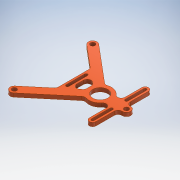
# Autodesk Inventor part: Pok Mk3 Base
Saved by Autodesk Inventor 2018.2 (Build 222227000, 227)
## iProperties
Created: 2018-02-12
Part Number: Pok Mk3 Base
Material: ABS Plastic
Document SubType Name: Modeling
Designer: Moochster
Density: 1.06 g/cm^3
Appearance: Smooth - Light Orange
Author: Moochster
Autodesk Inventor part; units mm, degrees
ref_plane "YZ Plane" through (0, 0, 0) normal (1, 0, 0) x (0, 1, 0)
ref_plane "XZ Plane" through (0, 0, 0) normal (0, 1, 0) x (-1, 0, 0)
ref_plane "XY Plane" through (0, 0, 0) normal (0, 0, 1) x (1, 0, 0)
sketch "Sketch1" plane through (0, 0, 0) normal (0, 0, 1) x (1, 0, 0)
  arc A0 (-5.6292, 10.5978) -> (-11.4143, 3.7034) centre (0, 0) ccw
  line L0 (11.1243, -4.5) -> (28, -4.5)
  arc A1 (28, -4.5) -> (28, 4.5) centre (28, 0) ccw
  line L1 (28, 4.5) -> (11.1243, 4.5)
  line L2 (0, 0) -> (28, 0) construction
  line L3 (0, 0) -> (-49.7929, 41.7812) construction
  line L4 (-5.6292, 10.5978) -> (-46.9003, 45.2284)
  arc A2 (-46.9003, 45.2284) -> (-52.6854, 38.334) centre (-49.7929, 41.7812) ccw
  line L5 (-52.6854, 38.334) -> (-11.4143, 3.7034)
  arc A3 (11.1243, 4.5) -> (-5.6292, 10.5978) centre (0, 0) ccw
  arc A4 (-11.4143, 3.7034) -> (-11.4143, -3.7034) centre (0, 0) ccw
  line L6 (-5.6292, -10.5978) -> (-46.9003, -45.2284)
  arc A5 (-52.6854, -38.334) -> (-46.9003, -45.2284) centre (-49.7929, -41.7812) ccw
  line L7 (-52.6854, -38.334) -> (-11.4143, -3.7034)
  arc A6 (-5.6292, -10.5978) -> (11.1243, 4.5) centre (0, 0) ccw
  arc A7 (-11.4143, -3.7034) -> (-5.6292, -10.5978) centre (0, 0) ccw
  circle A8 centre (28, 0) radius 2.5
  circle A9 centre (-49.7929, 41.7812) radius 2.5
  circle A10 centre (-49.7929, -41.7812) radius 2.5
  circle A11 centre (0, 0) radius 8.0875
  dimension "d0" = 24
  dimension "d5" = 5
  dimension "d6" = 2
  dimension "d7" = 28
  dimension "d8" = 65
  dimension "d9" = 140
  dimension "d10" = 5
  dimension "d11" = 2
  dimension "d12" = 5
  dimension "d13" = 16.175
  constraints: 19 point on circle, 16 end point, 12 centre point, 5 coincident, 5 symmetric about line, 4 parallel, 4 tangent, 1 horizontal, 1 other
  measures "d0" diameter of A0
  measures "d5" diameter of A8
  measures "d6" radial gap between concentric circles of A1 A8
  measures "d7" distance of L2.start L2.end
  measures "d8" distance of L2.start L3.end
  measures "d9" angle of L2 L3
  measures "d10" diameter of A9
  measures "d11" radial gap between concentric circles of A2 A9
  measures "d12" diameter of A10
  measures "d13" diameter of A11
extrude "Extrusion2" add sketch "Sketch1" along normal blind 4
sketch "Sketch2" plane through (0, 0, 0) normal (0, 0, 1) x (1, 0, 0)
  line L0 (-25, -10) -> (-25, 10) construction
  line L1 (-23.5, -10) -> (-23.5, 10)
  line L2 (-26.5, 10) -> (-26.5, -10)
  arc A0 (-26.5, -10) -> (-23.5, -10) centre (-25, -10) ccw
  arc A1 (-23.5, 10) -> (-26.5, 10) centre (-25, 10) ccw
  line L3 (20, 28) -> (20, 8) construction
  line L4 (18.5, 28) -> (18.5, 8)
  line L5 (21.5, 8) -> (21.5, 28)
  arc A2 (21.5, 28) -> (18.5, 28) centre (20, 28) ccw
  arc A3 (18.5, 8) -> (21.5, 8) centre (20, 8) ccw
  line L6 (20, -28) -> (20, -8) construction
  line L7 (21.5, -28) -> (21.5, -8)
  line L8 (18.5, -8) -> (18.5, -28)
  arc A4 (18.5, -28) -> (21.5, -28) centre (20, -28) ccw
  arc A5 (21.5, -8) -> (18.5, -8) centre (20, -8) ccw
  line L9 (11.1243, -4.5) -> (28, -4.5) projected
  line L10 (28, 4.5) -> (11.1243, 4.5) projected
  line L11 (-52.6854, 38.334) -> (-11.4143, 3.7034) projected
  line L12 (-11.4143, -3.7034) -> (-52.6854, -38.334) projected
  line L13 (16.5, 4.5) -> (16.5, 28)
  arc A6 (23.5, 28) -> (16.5, 28) centre (20, 28) ccw
  line L14 (23.5, 28) -> (23.5, 4.5)
  line L15 (16.5, -4.5) -> (16.5, -28)
  arc A7 (16.5, -28) -> (23.5, -28) centre (20, -28) ccw
  line L16 (23.5, -28) -> (23.5, -4.5)
  line L17 (-28.5, 18.04) -> (-28.5, -18.04)
  line L18 (-21.5, -12.1663) -> (-21.5, 12.1663)
  point P0 (0, 0)
  point P1 (-25, 0)
  point P2 (20, 18)
  point P3 (20, -18)
  dimension "d17" = 18
  dimension "d18" = 25
  dimension "d19" = 20
  dimension "d20" = 10
  dimension "d21" = 3
  dimension "d22" = 10
  dimension "d23" = 3
  dimension "d24" = 10
  dimension "d25" = 3
  dimension "d26" = 18
  dimension "d27" = 2
  dimension "d28" = 2
  dimension "d29" = 2
  dimension "d30" = 2
  constraints: 36 end point, 16 point on circle, 16 tangent, 9 point on line, 8 centre point, 5 parallel, 3 midpoint, 3 perpendicular, 3 vertical, 2 concentric, 1 horizontal alignment, 1 vertical alignment
  measures "d17" vertical distance of point (0, 0) point (20, -18)
  measures "d18" distance of point (0, 0) point (-25, 0)
  measures "d19" horizontal distance of point (0, 0) point (20, -18)
  measures "d20" distance of point (-25, 0) L0.end
  measures "d21" diameter of A1
  measures "d22" distance of point (20, 18) L3.end
  measures "d23" diameter of A3
  measures "d24" distance of point (20, -18) L6.end
  measures "d25" diameter of A5
  measures "d26" vertical distance of point (0, 0) point (20, 18)
  measures "d27" radial gap between concentric circles of A2 A6
  measures "d28" radial gap between concentric circles of A4 A7
  measures "d29" distance between parallel lines of L1 L18
  measures "d30" distance between parallel lines of L17 L2
extrude "Extrusion3" add sketch "Sketch2" along normal up to surface (4 mm away)
fillet "Fillet1" radius 4 14 edges at (23.5, -4.5, 2) (23.5, 4.5, 2) (16.5, 4.5, 2) (11.1243, -4.5, 2) (11.1243, 4.5, 2) (-5.6292, 10.5978, 2) (-5.6292, -10.5978, 2) (-21.5, 12.1663, 2) (-21.5, -12.1663, 2) (-28.5, -18.04, 2) (-28.5, 18.04, 2) (-11.4143, 3.7034, 2) (-11.4143, -3.7034, 2) (16.5, -4.5, 2)
body "Solid2"
